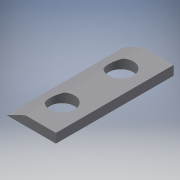
# Autodesk Inventor part: top_slant
Saved by Autodesk Inventor 2017 (Build 210142000, 142)
## iProperties
Created: 2019-03-22
Part Number: top_slant
Material: Generic
Document SubType Name: Modeling
Designer: Mitch
Density: 1 g/cm^3
Appearance: Default
Author: Mitch
Autodesk Inventor part; units mm, degrees
ref_plane "YZ Plane" through (0, 0, 0) normal (1, 0, 0) x (0, 1, 0)
ref_plane "XZ Plane" through (0, 0, 0) normal (0, 1, 0) x (-1, 0, 0)
ref_plane "XY Plane" through (0, 0, 0) normal (0, 0, 1) x (1, 0, 0)
sketch "Sketch1" plane through (0, 0, 0) normal (0, 1, 0) x (-1, 0, 0)
  line L0 (0, 0) -> (101.6, 0)
  line L1 (101.6, 0) -> (101.6, -241.3)
  line L2 (101.6, -241.3) -> (0, -241.3)
  line L3 (0, -241.3) -> (0, 0)
  dimension "d0" = 101.6
  dimension "d1" = 241.3
  constraints: 8 end point, 2 parallel, 1 horizontal, 1 perpendicular
  measures "d0" distance of L1.end L2.end
  measures "d1" distance of L0.end L1.end
extrude "Extrusion1" add sketch "Sketch1" along normal blind 19.05
hole "Hole1" at (-47.625, 0, -180.975) direction (0, 1, 0) diameter 50.8 end through all
hole "Hole2" at (-47.625, 0, -60.325) direction (0, 1, 0) diameter 50.8 end through all
sketch "Sketch3" plane through (-101.6, 0, 0) normal (0, 0, 1) x (1, 0, 0)
  line L0 (18.0708, 8.9693) -> (0.9487, 0.6183) projected
  line L1 (0.9487, 0.6183) -> (0, 0.1556)
  line L2 (0, 0) -> (0, 19.05) projected
  line L3 (18.0708, 8.9693) -> (38.7393, 19.05)
  line L4 (0, 19.05) -> (101.6, 19.05) projected
  line L5 (38.7393, 19.05) -> (0, 19.05)
  point P0 (101.6, 0)
  constraints: 6 end point, 3 point on line, 1 horizontal
extrude "Extrusion3" cut sketch "Sketch3" against normal blind 241.3
body "Solid1"
